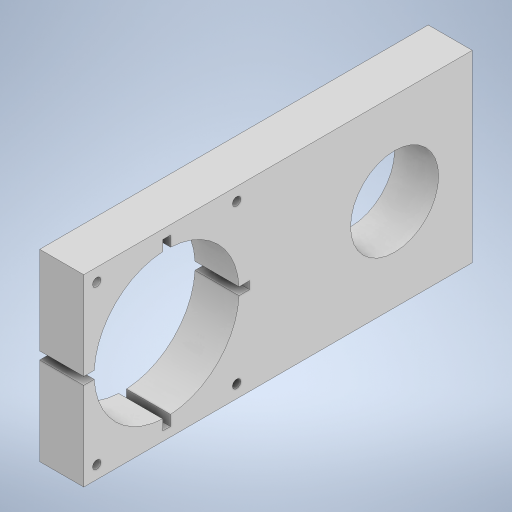
# Autodesk Inventor part: Joint2_Gear_Housing
Saved by Autodesk Inventor 2023 (Build 270158030, 158C)
## iProperties
Created: 2022-06-16
Part Number: Joint2_Gear_Housing
Material: Generic
Document SubType Name: Modeling
Designer: Mlees
Density: 1 g/cm^3
Appearance: Default
Author: Mlees
Autodesk Inventor part; units mm, degrees
ref_plane "YZ Plane" through (0, 0, 0) normal (1, 0, 0) x (0, 1, 0)
ref_plane "XZ Plane" through (0, 0, 0) normal (0, 1, 0) x (-1, 0, 0)
ref_plane "XY Plane" through (0, 0, 0) normal (0, 0, 1) x (1, 0, 0)
sketch "Sketch1" plane through (0, 0, 0) normal (1, 0, 0) x (0, 1, 0)
  line L0 (71, 0) -> (71, -150)
  line L1 (71, -150) -> (0, -150)
  line L2 (0, -150) -> (0, 0)
  line L3 (35.5, 0) -> (37, 0)
  line L4 (35.5, 0) -> (34, 0)
  line L5 (34, 0) -> (34, -4.0402)
  line L6 (37, 0) -> (37, -4.0402)
  line L7 (3.5, -30.5) -> (7.5402, -30.5)
  line L8 (3.5, -32) -> (3.5, -30.5)
  line L9 (3.5, -32) -> (3.5, -33.5)
  line L10 (3.5, -33.5) -> (7.5402, -33.5)
  line L11 (34, -64) -> (34, -59.9598)
  line L12 (35.5, -64) -> (34, -64)
  line L13 (35.5, -64) -> (37, -64)
  line L14 (37, -64) -> (37, -59.9598)
  line L15 (67.5, -33.5) -> (63.4598, -33.5)
  line L16 (67.5, -32) -> (67.5, -33.5)
  line L17 (67.5, -32) -> (67.5, -30.5)
  line L18 (67.5, -30.5) -> (63.4598, -30.5)
  arc A0 (63.4598, -30.5) -> (37, -4.0402) centre (35.5, -32) ccw
  arc A1 (37, -59.9598) -> (63.4598, -33.5) centre (35.5, -32) ccw
  arc A2 (34, -4.0402) -> (7.5402, -30.5) centre (35.5, -32) ccw
  arc A3 (7.5402, -33.5) -> (34, -59.9598) centre (35.5, -32) ccw
  line L19 (0, 0) -> (34, 0)
  line L20 (37, 0) -> (71, 0)
  circle A4 centre (35.5, -120) radius 17
  dimension "d0" = 71
  dimension "d1" = 150
  dimension "d2" = 1.5
  dimension "d8" = 360
  dimension "d13" = 34
  constraints: 42 end point, 8 point on circle, 5 centre point, 3 equal length, 1 horizontal, 1 perpendicular, 37 other
  measures "d0" distance of L0.end L1.end
  measures "d1" distance of L0.start L0.end
  measures "d2" distance of L3.start L3.end
  measures "d13" diameter of A4
extrude "Extrusion2" add sketch "Sketch1" along normal blind 17 contours L0 L1 L2 L19 L5 A2 L7 L8 L9 L10 A3 L11 L12 L13 L14 A1 L15 L16 L17 L18 A0 L6 L20
sketch "Sketch2" plane through (17, 0, 0) normal (1, 0, 0) x (0, 0, -1)
  line L0 (0, 0) -> (5, 0)
  line L1 (0, 0) -> (150, 0) projected
  line L2 (150, 71) -> (0, 71) projected
  line L3 (5, 71) -> (10, 71) construction
  point P0 (5, 5)
  point P1 (5, 66)
  point P2 (59, 66)
  point P3 (59, 5)
  constraints: 4 end point, 2 point on line, 1 horizontal
hole "Hole1" at (17, 5, -5) at (17, 66, -5) at (17, 66, -59) at (17, 5, -59) direction (-1, 0, 0) diameter 3.25 end through all
body "Solid2"
